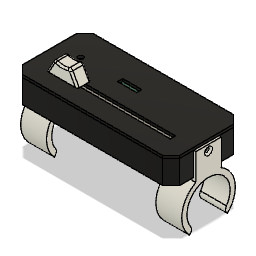
Hydroponics_Fan_Controller (Autodesk Fusion 360 design; units mm, degrees)
Autodesk Fusion 360 part; units mm, degrees
note: some values were not read from the file. Set by a fixed rule: which sketch regions a step uses.
sketch "Sketch1" plane through (0, 0, 0) normal (0, 1, 0) x (1, 0, 0)
  line L0 (0, 0) -> (85, 0)
  line L1 (85, 0) -> (85, -35)
  line L2 (85, -35) -> (0, -35)
  line L3 (0, -35) -> (0, 0)
  dimension "d1" = 85
  dimension "d2" = 35
  constraint horizontal L0
  constraint vertical L1
  constraint horizontal L2
  constraint vertical L3
  constraint coincident L0.start L3.end
  measures "d1" distance of L0.start L0.end
  measures "d2" distance of L0.start L2.end
extrude "Extrude1" add sketch "Sketch1" along normal blind 1.6 makes body 1
sketch "Sketch2" plane through (0, 1.6, 0) normal (0, 1, 0) x (-1, 0, 0)
  line L0 (0, 35) -> (-85, 35)
  line L1 (-85, 35) -> (-85, 0)
  line L2 (-85, 0) -> (0, 0)
  line L3 (0, 0) -> (0, 35)
  line L4 (0, 35) -> (0, 32)
  line L5 (0, 32) -> (0, 20)
  line L6 (0, 35) -> (-5, 35)
  line L7 (-5, 35) -> (-82, 35)
  line L8 (0, 32) -> (-82, 32)
  line L9 (-82, 32) -> (-5, 32)
  line L10 (-5, 32) -> (-5, 20)
  line L11 (-5, 20) -> (-82, 20)
  line L12 (-82, 20) -> (-82, 32)
  dimension "d5" = 3
  dimension "d6" = 12
  dimension "d7" = 5
  dimension "d8" = 77
  constraint coincident L0.start L3.end
  constraint perpendicular L2 L4
  constraint parallel L3 L5
  constraint perpendicular L4 L6
  constraint perpendicular L1 L7
  constraint perpendicular L4 L8
  constraint horizontal L9
  constraint vertical L10
  constraint horizontal L11
  constraint vertical L12
  measures "d5" distance of L0.start L4.end
  measures "d6" distance of L4.end L5.end
  measures "d7" distance of L0.start L6.end
  measures "d8" distance of L6.end L7.end
extrude "Extrude2" add sketch "Sketch2" along normal blind 10 contours L8 L9 L10 L11 L12 bodies 1
sketch "Sketch3" plane through (0, 11.6, 0) normal (0, 1, 0) x (-1, 0, 0)
  line L0 (-82, 20) -> (-5, 20)
  line L1 (-5, 20) -> (-5, 32)
  line L2 (-5, 32) -> (-82, 32)
  line L3 (-82, 32) -> (-82, 20)
  line L4 (-5, 26) -> (-10, 26)
  line L5 (-10, 26) -> (-10, 24.5)
  line L6 (-82, 26) -> (-77, 26)
  line L7 (-77, 26) -> (-77, 27.5)
  line L8 (-10, 24.5) -> (-77, 24.5)
  line L9 (-77, 24.5) -> (-77, 27.5)
  line L10 (-77, 27.5) -> (-10, 27.5)
  line L11 (-10, 27.5) -> (-10, 24.5)
  line L12 (-13, 26) -> (-13, 25.25)
  line L13 (-13, 25.25) -> (-20.5, 25.25)
  line L14 (-20.5, 25.25) -> (-20.5, 26.75)
  line L15 (-20.5, 26.75) -> (-13, 26.75)
  line L16 (-13, 26.75) -> (-13, 25.25)
  dimension "d11" = 5
  dimension "d12" = 1.5
  dimension "d13" = 5
  dimension "d14" = 1.5
  dimension "d15" = 0.75
  dimension "d16" = 7.5
  dimension "d17" = 1.5
  constraint midpoint L1 L4.start
  constraint perpendicular L1 L4
  constraint perpendicular L4 L5
  constraint midpoint L3 L6.start
  constraint perpendicular L3 L6
  constraint perpendicular L6 L7
  constraint horizontal L8
  constraint vertical L9
  constraint horizontal L10
  constraint vertical L11
  constraint perpendicular L8 L12
  constraint horizontal L13
  constraint vertical L14
  constraint horizontal L15
  constraint vertical L16
  measures "d11" distance of L4.start L4.end
  measures "d12" distance of L4.end L5.end
  measures "d13" distance of L6.start L6.end
  measures "d14" distance of L6.end L7.end
  measures "d15" distance of L12.start L12.end
  measures "d16" distance of L12.end L13.end
  measures "d17" distance of L12.end L15.end
extrude "Extrude3" cut sketch "Sketch3" against normal blind 5 contours L5 L7 L8 L9 L10 L11 bodies 1
extrude "Extrude4" add 1 faces at (18, 11.6, 26.25) along direction (0, 1, 0) blind 8 on bodies 1 bodies 1
sketch "Sketch4" plane through (0, 0, 26.75) normal (0, 0, 1) x (1, 0, 0)
  line L0 (13, 19.6) -> (13, 6.6)
  line L1 (13, 6.6) -> (20.5, 6.6)
  line L2 (20.5, 6.6) -> (20.5, 19.6)
  line L3 (20.5, 19.6) -> (13, 19.6)
sketch "Sketch5" plane through (0, 0, 0) normal (0, 1, 0) x (1, 0, 0)
  line L0 (85, 0) -> (0, 0)
  line L1 (0, 0) -> (0, -35)
  line L2 (0, -35) -> (85, -35)
  line L3 (85, -35) -> (85, 0)
  line L4 (-0.15, -35.15) -> (85.15, -35.15)
  line L5 (85.15, -35.15) -> (85.15, 0.15)
  line L6 (85.15, 0.15) -> (-0.15, 0.15)
  line L7 (-0.15, 0.15) -> (-0.15, -35.15)
  line L8 (-3, -38) -> (88, -38)
  line L9 (88, -38) -> (88, 3)
  line L10 (88, 3) -> (-3, 3)
  line L11 (-3, 3) -> (-3, -38)
  dimension "d22" = 0.15
  dimension "d23" = 3
extrude "Extrude5" add sketch "Sketch5" along normal up to surface (11.6 mm away) separate body contours L8 L9 L10 L11 makes body 2
extrude "Extrude6" add sketch "Sketch5" against normal blind 2 separate body contours L0 L1 L2 L3 | L4 L5 L6 L7 | L8 L9 L10 L11 makes body 3
combine "Combine1" operation add target body 2 tool bodies 3
sketch "Sketch6" plane through (0, 11.6, 0) normal (0, 1, 0) x (-1, 0, 0)
  line L0 (-85.15, 35.15) -> (0.15, 35.15)
  line L1 (0.15, 35.15) -> (0.15, -0.15)
  line L2 (0.15, -0.15) -> (-85.15, -0.15)
  line L3 (-85.15, -0.15) -> (-85.15, 35.15)
  line L4 (-88, -3) -> (3, -3)
  line L5 (3, -3) -> (3, 38)
  line L6 (3, 38) -> (-88, 38)
  line L7 (-88, 38) -> (-88, -3)
  line L8 (3, -3) -> (-88, -3)
  line L9 (3, 38) -> (3, -3)
  line L10 (-88, 38) -> (3, 38)
  line L11 (-88, -3) -> (-88, 38)
  line L12 (-77, 24.5) -> (-77, 27.5)
  line L13 (-10, 24.5) -> (-77, 24.5)
  line L14 (-77, 27.5) -> (-10, 27.5)
  line L15 (-10, 27.5) -> (-10, 24.5)
  line L16 (0.15, -0.15) -> (0.15, 35.15)
  line L17 (-85.15, -0.15) -> (0.15, -0.15)
  line L18 (-85.15, 35.15) -> (-85.15, -0.15)
  line L19 (0.15, 35.15) -> (-85.15, 35.15)
  line L20 (-85, 0) -> (-85, 35)
  line L21 (-85, 35) -> (0, 35)
  line L22 (0, 35) -> (0, 0)
  line L23 (0, 0) -> (-85, 0)
  line L24 (-83.15, 1.85) -> (-83.15, 33.15)
  line L25 (-83.15, 33.15) -> (-1.85, 33.15)
  line L26 (-1.85, 33.15) -> (-1.85, 1.85)
  line L27 (-1.85, 1.85) -> (-83.15, 1.85)
  line L28 (-1.85, 1.85) -> (-1.85, -0.15)
  line L29 (-1.85, -0.15) -> (-1.85, 33.15)
  line L30 (-1.85, 33.15) -> (-1.85, 36)
  line L31 (-83.15, 1.85) -> (-83.15, -1)
  line L32 (-83.15, 33.15) -> (-83.15, 36)
  line L33 (-33, 11) -> (-44, 11)
  line L34 (-44, 11) -> (-44, 14)
  line L35 (-44, 14) -> (-33, 14)
  line L36 (-33, 14) -> (-33, 11)
  circle A0 centre (-10.1225, 12.5) radius 1.5
  dimension "d28" = 0.15
  dimension "d29" = 2
  dimension "d82" = 11
  dimension "d83" = 3
  dimension "d84" = 3
  constraint coincident L17 L28.end
  constraint perpendicular L17 L28
  constraint perpendicular L19 L30
  constraint perpendicular L17 L31
  constraint perpendicular L19 L32
  constraint horizontal L33
  constraint vertical L34
  constraint horizontal L35
  constraint vertical L36
  measures "d82" distance of L33.start L33.end
  measures "d83" distance of L33.start L35.end
  measures "d84" diameter of A0
extrude "Extrude7" add sketch "Sketch6" against normal blind 7 separate body contours L20 L21 L23 L24 L31 L32 | L21 L22 L23 L26 L28 L29 L30 makes body 4 at (0, 9.2667, 23.3333) makes body 5 at (83.15, 9.2667, 11.6667)
extrude "Extrude8" add sketch "Sketch6" along normal blind 1.5 separate body contours L0 L2 L3 L17 L18 L19 L20 L21 L23 L31 L32 | L0 L19 L21 L30 L32 | L0 L1 L2 L16 L17 L19 L21 L22 L23 L28 L29 L30 | L20 L21 L23 L24 L31 L32 | L21 L25 L30 L32 | L2 L17 L23 L28 L29 L31 | L21 L22 L23 L26 L28 L29 L30 | L24 L25 L26 L27 L29 | L23 L27 L28 L29 L31 | L4 L5 L6 L7 L8 L9 L10 L11 makes body 6
combine "Combine2" operation add target body 4 tool bodies 5 6
ref_plane "WorkPlane1" through (16.75, 13.1, 26) normal (0, 0, 1) x (-1, 0, 0)
sketch "Sketch7" plane through (16.75, 13.1, 26) normal (0, 0, 1) x (1, 0, 0)
  line L0 (-3.75, -6.5) -> (-3.75, 6.5)
  line L1 (-3.75, 6.5) -> (3.75, 6.5)
  line L2 (3.75, 6.5) -> (3.75, -6.5)
  line L3 (-3.9, -6.5) -> (-3.9, 6.65)
  line L4 (-3.9, 6.65) -> (3.9, 6.65)
  line L5 (3.9, 6.65) -> (3.9, -6.5)
  circle A0 centre (-3.9, 6.65) radius 1.5
  circle A1 centre (3.9, 6.65) radius 1.5
  line L6 (-3.75, 7.5) -> (3.75, 7.5)
  spline S0 degree 5 poles (3.4308, 8.0747) (3.2935, 8.0311) (3.0191, 7.9478) (2.6074, 7.8341) (2.0585, 7.7058) (1.3723, 7.5867) (0.6862, 7.5127) (0, 7.4874) (-0.6862, 7.5127) (-1.3723, 7.5867) (-2.0585, 7.7058) (-2.6074, 7.8341) (-3.0191, 7.9478) (-3.2935, 8.0311) (-3.4308, 8.0747) knots 0 0 0 0 0 0 0.1 0.2 0.3 0.4 0.5 0.6 0.7 0.8 0.9 1 1 1 1 1 1
  line L7 (-3.9, 6.65) -> (-3.9, 0.65)
  line L8 (-3.9, 0.65) -> (-8.9, 0.65)
  line L9 (0, 7.5) -> (0, 0)
  line L10 (-8.9, 0.65) -> (-5.2153, 7.3711)
  line L11 (3.9, 0.65) -> (8.9, 0.65)
  line L12 (3.75, 6.5) -> (-3.75, 6.5)
  circle A2 centre (-3.9, 6.65) radius 1.5
  line L13 (3.75, 7.5) -> (-3.75, 7.5)
  spline S1 degree 5 poles (-3.4308, 8.0747) (-3.2935, 8.0311) (-3.0191, 7.9478) (-2.6074, 7.8341) (-2.0585, 7.7058) (-1.3723, 7.5867) (-0.6862, 7.5127) (0, 7.4874) (0.6862, 7.5127) (1.3723, 7.5867) (2.0585, 7.7058) (2.6074, 7.8341) (3.0191, 7.9478) (3.2935, 8.0311) (3.4308, 8.0747) knots 0 0 0 0 0 0 0.1 0.2 0.3 0.4 0.5 0.6 0.7 0.8 0.9 1 1 1 1 1 1
  line L14 (4.12, 8.2936) -> (2.7415, 7.8558)
  line L15 (-2.7415, 7.8558) -> (-4.12, 8.2936)
  line L16 (-4.12, 8.2936) -> (-2.7415, 7.8558)
  line L17 (2.7415, 7.8558) -> (4.12, 8.2936)
  line L18 (8.9, 0.65) -> (5.2153, 7.3711)
  line L19 (3.9, 6.65) -> (-3.9, 6.65)
  circle A3 centre (3.9, 6.65) radius 1.5
  line L20 (3.9, 6.65) -> (3.9, 0.65)
  point P0 (0, 7.5)
  point P1 (0, 7.5)
  point P2 (0, 7.5)
  dimension "d34" = -0.15
  dimension "d35" = 3
  dimension "d36" = 3
  dimension "d37" = -1
  dimension "d38" = 6
  dimension "d39" = 5
  constraint coincident L3.end L4.start
  constraint coincident L4.end L5.start
  constraint coincident A1 S0.start
  constraint midpoint L6 P2
  constraint coincident A0 S0.end
  constraint perpendicular L4 L7
  constraint perpendicular L3 L8
  constraint coincident P2 P1
  constraint coincident L9.end origin
  constraint perpendicular L1 L9
  constraint coincident A0 L10.end
  constraint tangent A0 L10
  constraint midpoint S0.start L14
  constraint midpoint S0.end L15
  constraint symmetric L0.end L9 L1.end
  constraint symmetric L1.end L9 L0.end
  constraint symmetric L3.end L9 L4.end
  constraint symmetric L4.end L9 L3.end
  constraint symmetric A0 L9 A3
  constraint symmetric A1 L9 A2
  constraint symmetric L6.start L9 L6.end
  constraint symmetric L6.end L9 L6.start
  constraint symmetric S0.start L9 S0.end
  constraint symmetric P2 L9 P1
  constraint symmetric S0.end L9 S0.start
  constraint symmetric L7.end L9 L11.start
  constraint symmetric L8.end L9 L11.end
  constraint symmetric L9 L10.end L18.end
  constraint symmetric L9 L14.start L15.end
  constraint symmetric L9 L14.end L15.start
  constraint symmetric L9 L15.start L14.end
  constraint symmetric L9 L15.end L14.start
  measures "d35" diameter of A0
  measures "d36" diameter of A1
  measures "d38" distance of L3.end L7.end
  measures "d39" distance of L7.end L8.end
extrude "Extrude9" add sketch "Sketch7" along normal mid plane 1.8 separate body contours L3 L4 A0 L7 A2 L19 | L3 A0 L7 L8 L10 A2 | L4 A0 L6 L9 A2 L13 L19 | A0 L6 S0 A2 L13 S1 | L4 A1 L6 L9 L13 L19 A3 | A1 L6 S0 L13 S1 A3 | L4 L5 A1 L19 A3 L20 | L5 A1 L11 L18 A3 L20 makes body 7
sketch "Sketch8" plane through (0, 0, 26.9) normal (0, 0, 1) x (1, 0, 0)
  line L0 (12.85, 19.75) -> (20.65, 19.75)
  line L1 (20.65, 19.75) -> (20.65, 13.75)
  line L2 (20.65, 13.75) -> (25.65, 13.75)
  line L3 (25.65, 13.75) -> (21.9653, 20.4711)
  arc A0 (21.9653, 20.4711) -> (20.1808, 21.1747) centre (20.65, 19.75) ccw
  spline S0 degree 5 poles (20.1808, 21.1747) (20.0435, 21.1311) (19.7691, 21.0478) (19.3574, 20.9341) (18.8085, 20.8058) (18.1223, 20.6867) (17.4362, 20.6127) (16.75, 20.5874) (16.0638, 20.6127) (15.3777, 20.6867) (14.6915, 20.8058) (14.1426, 20.9341) (13.7309, 21.0478) (13.4565, 21.1311) (13.3192, 21.1747) knots -1 -1 -1 -1 -1 -1 -0.9 -0.8 -0.7 -0.6 -0.5 -0.4 -0.3 -0.2 -0.1 0 0 0 0 0 0
  arc A1 (13.3192, 21.1747) -> (11.5347, 20.4711) centre (12.85, 19.75) ccw
  line L4 (11.5347, 20.4711) -> (7.85, 13.75)
  line L5 (7.85, 13.75) -> (12.85, 13.75)
  line L6 (12.85, 13.75) -> (12.85, 19.75)
  line L7 (11.5347, 20.4711) -> (7.85, 13.75)
  line L8 (12.85, 13.75) -> (20.65, 13.75)
  constraint coincident L5.end L6.start
  constraint coincident L1.end L2.start
extrude "Extrude10" add sketch "Sketch8" along normal blind 3 bodies 7
mirror "Mirror1" about plane through (16.75, 13.1, 26) normal (0, 0, 1) of "Extrude10"
chamfer "Chamfer1" distance 5 angle 45 8 edges at (-3, 4.8, -3) (-3, 4.8, 38) (88, 4.8, 38) (88, 4.8, -3) (-3, 12.35, -3) (-3, 12.35, 38) (88, 12.35, 38) (88, 12.35, -3) on bodies 2 4
sketch "Sketch9" plane through (88, 0, 0) normal (1, 0, 0) x (0, 0, -1)
  line L0 (-2, -2) -> (-2, 11.6)
  line L1 (-2, 11.6) -> (-33, 11.6)
  line L2 (-33, 11.6) -> (-33, -2)
  line L3 (-33, -2) -> (-2, -2)
  line L4 (0, 4.6) -> (-35, 4.6)
  line L5 (-2, 11.6) -> (-33, 11.6)
  line L6 (-17.5, 11.6) -> (-17.5, 8.1)
  circle A0 centre (-17.5, 8.1) radius 0.8
  circle A1 centre (-17.5, 8.1) radius 1.25
  dimension "d47" = 3.5
  dimension "d48" = 1.6
  dimension "d49" = 2.5
  constraint midpoint L1 L6.start
  constraint perpendicular L4 L6
  constraint coincident L6.end A0.centre
  constraint concentric A0 A1
  measures "d47" distance of L6.start L6.end
  measures "d48" diameter of A0
  measures "d49" diameter of A1
extrude "Extrude11" cut sketch "Sketch9" against normal up to surface (88 mm away) contours A0 bodies 4
extrude "Extrude12" cut sketch "Sketch9" against normal up to surface (91 mm away) contours A0 | A1 bodies 2
fillet "Fillet1" radius 1 10 edges at (12.2998, 21.1454, 29.9) (9.6923, 17.1105, 29.9) (16.75, 20.6, 29.9) (23.8077, 17.1105, 29.9) (21.2002, 21.1454, 29.9) (23.8077, 17.1105, 22.1) (21.2002, 21.1454, 22.1) (16.75, 20.6, 22.1) (12.2998, 21.1454, 22.1) (9.6923, 17.1105, 22.1) on bodies 7
sketch "Sketch10" plane through (-3, 0, 0) normal (-1, 0, 0) x (0, 0, 1)
  circle A0 centre (17.5, 8.1) radius 1.25
  line L0 (33, -2) -> (33, 11.6)
  line L1 (33, 11.6) -> (2, 11.6)
  line L2 (2, 11.6) -> (2, -2)
  line L3 (2, -2) -> (33, -2)
  line L4 (33, 11.6) -> (2, 11.6)
  circle A1 centre (17.5, 8.1) radius 1.25
  line L5 (17.5, 11.6) -> (10, 11.6)
  line L6 (10, 11.6) -> (25, 11.6)
  line L7 (25, 11.6) -> (25, -2)
  line L8 (25, -2) -> (10, -2)
  line L9 (10, -2) -> (10, 11.6)
  line L10 (10.15, -2) -> (10.15, 11.45)
  line L11 (10.15, 11.45) -> (24.85, 11.45)
  line L12 (24.85, 11.45) -> (24.85, -2)
  dimension "d57" = 15
  dimension "d58" = 0.15
  constraint midpoint L4 L5.start
  constraint coincident L4 L5.end
  constraint parallel L4 L5
  constraint horizontal L6
  constraint vertical L7
  constraint horizontal L8
  constraint vertical L9
  measures "d57" distance of L5.end L6.end
extrude "Extrude13" cut sketch "Sketch10" against normal blind 1 contours L1 L3 L4 L5 L6 L7 L8 L9 L10 L11 L12 | L3 L8 L10 L11 L12 bodies 2
extrude "Extrude14" add sketch "Sketch10" along normal blind 1.15 and the other way blind 0.85 separate body contours L3 L8 L10 L11 L12 makes body 8
sketch "Sketch11" plane through (-4.15, 0, 0) normal (-1, 0, 0) x (0, 0, 1)
  circle A0 centre (17.5, 8.1) radius 1.25
  line L0 (24.85, 11.45) -> (10.15, 11.45)
  line L1 (10.15, 11.45) -> (10.15, -2)
  line L2 (10.15, -2) -> (24.85, -2)
  line L3 (24.85, -2) -> (24.85, 11.45)
  line L4 (10.15, -2) -> (24.85, -2)
  line L5 (24.85, -2) -> (24.85, -4)
  line L6 (24.85, -4) -> (10.15, -4)
  line L7 (10.15, -4) -> (10.15, -2)
  circle A1 centre (17.5, -17.6465) radius 15.5
  circle A2 centre (17.5, -17.6465) radius 12.5
  line L8 (17.5, -17.6465) -> (6.5398, -28.6067)
  line L9 (17.5, -17.6465) -> (33, -17.6465) construction
  line L10 (17.5, -17.6465) -> (28.4602, -28.6067)
  line L11 (17.5, -17.6465) -> (33, -17.6465) construction
  line L12 (10.15, -2.15) -> (24.85, -2.15)
  dimension "d66" = 2
  dimension "d67" = 31
  dimension "d68" = 25
  dimension "d69" = 135
  dimension "d70" = 45
  dimension "d71" = 0.15
  constraint horizontal L4
  constraint vertical L5
  constraint horizontal L6
  constraint vertical L7
  constraint coincident L1.end L2.start
  constraint coincident L6.end A1
  constraint coincident L5.end A1
  constraint concentric A1 A2
  constraint horizontal L9
  constraint coincident A1.centre A2.centre
  constraint horizontal L11
  measures "d66" distance of L1.end L6.end
  measures "d67" diameter of A1
  measures "d68" diameter of A2
  measures "d69" angle of L8 L9
  measures "d70" angle of L10 L11
extrude "Extrude15" add sketch "Sketch11" against normal blind 2 contours L2 L4 L5 L7 A1 L12 | A1 L12 bodies 8
extrude "Extrude16" add sketch "Sketch11" against normal blind 15 contours L5 A1 L12 | L7 A1 L12 | L6 A1 A2 L8 L10 | L6 A1 L12 bodies 8
fillet "Fillet2" radius 3 2 edges at (3.35, -26.4854, 26.3388) (3.35, -26.4854, 8.6612) on bodies 8
chamfer "Chamfer3" distance 1 angle 45 1 edges at (-4.15, 8.552, 16.3346) on bodies 8
ref_plane "WorkPlane2" through (42.5, 4.8, 29) normal (-1, 0, 0) x (0, 0, 1)
mirror "Mirror2" about plane through (42.5, 4.8, 29) normal (-1, 0, 0) of "Extrude13"
mirror "Mirror3" about plane through (42.5, 4.8, 29) normal (-1, 0, 0) of bodies 8 makes body 9
equation "d8 = 82 mm - 5 mm"
equation "d15 = ( 1.5 / 2 ) * 1 mm"
equation "d40 = 1.5 mm + 0.3 mm"
equation "d47 = ( 7 / 2 ) * 1 mm"
equation "d61 = 2 mm - 0.85 mm"
equation "d67 = 25 mm + 6 mm"
named bodies: "Circuit Board", "Case Bottom", "Case Top", "Slider Cap", "Clip 1", "Clip 2"
